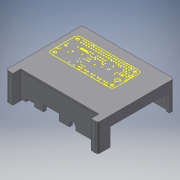
# Autodesk Inventor part: upperPiCase_small
Saved by Autodesk Inventor 2017 (Build 210142000, 142)
## iProperties
Created: 2017-11-29
Part Number: upperPiCase_small
Material: Generic
Document SubType Name: Modeling
Designer: Paolo
Density: 1 g/cm^3
Appearance: Default
Author: Paolo
Autodesk Inventor part; units mm, degrees
ref_plane "YZ Plane" through (0, 0, 0) normal (1, 0, 0) x (0, 1, 0)
ref_plane "XZ Plane" through (0, 0, 0) normal (0, 1, 0) x (-1, 0, 0)
ref_plane "XY Plane" through (0, 0, 0) normal (0, 0, 1) x (1, 0, 0)
ref_plane "Work Plane5" through (0, 0, 0) normal (0, 0, 1) x (1, 0, 0)
sketch "Sketch1" plane through (0, 0, 0) normal (0, 0, 1) x (1, 0, 0)
  line L0 (74.5037, -44.5224) -> (71.3037, -44.5224) projected
  line L1 (71.3037, -44.5224) -> (71.3037, -29.3224) projected
  line L2 (71.3037, -29.3224) -> (74.5037, -29.3224) projected
  line L3 (74.5037, -44.5224) -> (74.5037, -29.3224) projected
  line L4 (74.5037, 13.2776) -> (74.5037, 28.4776) projected
  line L5 (74.5037, 13.2776) -> (71.3037, 13.2776) projected
  line L6 (71.3037, 13.2776) -> (71.3037, 28.4776) projected
  line L7 (71.3037, 28.4776) -> (74.5037, 28.4776) projected
  circle A0 centre (-7.1663, -32.5224) radius 1.1 projected
  line L8 (-11.2963, 13.2776) -> (-14.4963, 13.2776) projected
  line L9 (-14.4963, 28.4776) -> (-14.4963, 13.2776) projected
  line L10 (-14.4963, 28.4776) -> (-11.2963, 28.4776) projected
  line L11 (-11.2963, 28.4776) -> (-11.2963, 13.2776) projected
  line L12 (-11.2963, -44.5224) -> (-14.4963, -44.5224) projected
  line L13 (-14.4963, -29.3224) -> (-14.4963, -44.5224) projected
  line L14 (-14.4963, -29.3224) -> (-11.2963, -29.3224) projected
  line L15 (-11.2963, -29.3224) -> (-11.2963, -44.5224) projected
  circle A1 centre (-7.1663, 16.4776) radius 1.1 projected
  arc A2 (-9.5963, 14.7183) -> (-9.5963, 18.2369) centre (-7.1663, 16.4776) ccw projected
  line L16 (-9.5963, 27.9776) -> (-9.5963, 18.2369) projected
  line L17 (69.6037, 27.9776) -> (-9.5963, 27.9776) projected
  line L18 (69.6037, 27.9776) -> (69.6037, 11.2776) projected
  line L19 (69.6037, 11.2776) -> (71.5037, 11.2776) projected
  line L20 (71.5037, 11.2776) -> (71.5037, -27.3224) projected
  line L21 (71.5037, -27.3224) -> (69.6037, -27.3224) projected
  line L22 (69.6037, -36.0224) -> (69.6037, -27.3224) projected
  line L23 (69.6037, -38.5224) -> (69.6037, -36.0224) projected
  line L24 (69.6037, -46.5224) -> (69.6037, -38.5224) projected
  line L25 (74.5037, -46.5224) -> (69.6037, -46.5224) projected
  arc A3 (74.5037, -46.5224) -> (76.5037, -44.5224) centre (74.5037, -44.5224) ccw projected
  line L26 (76.5037, -44.5224) -> (76.5037, 28.4776) projected
  arc A4 (76.5037, 28.4776) -> (74.5037, 30.4776) centre (74.5037, 28.4776) ccw projected
  line L27 (74.5037, 30.4776) -> (-14.4963, 30.4776) projected
  arc A5 (-14.4963, 30.4776) -> (-16.4963, 28.4776) centre (-14.4963, 28.4776) ccw projected
  line L28 (-16.4963, -44.5224) -> (-16.4963, 28.4776) projected
  arc A6 (-16.4963, -44.5224) -> (-14.4963, -46.5224) centre (-14.4963, -44.5224) ccw projected
  line L29 (-14.4963, -46.5224) -> (-9.5963, -46.5224) projected
  line L30 (-9.5963, -38.5224) -> (-9.5963, -46.5224) projected
  line L31 (-9.5963, -36.0224) -> (-9.5963, -38.5224) projected
  line L32 (-9.5963, -34.2817) -> (-9.5963, -36.0224) projected
  arc A7 (-9.5963, -34.2817) -> (-9.5963, -30.7631) centre (-7.1663, -32.5224) ccw projected
  line L33 (-9.5963, -27.3224) -> (-9.5963, -30.7631) projected
  line L34 (-13.4963, -27.3224) -> (-9.5963, -27.3224) projected
  line L35 (-13.4963, -27.3224) -> (-13.4963, 11.2776) projected
  line L36 (-13.4963, 11.2776) -> (-9.5963, 11.2776) projected
  line L37 (-9.5963, 14.7183) -> (-9.5963, 11.2776) projected
  line L38 (69.6037, -38.5224) -> (-9.5963, -38.5224) projected
  line L39 (-9.5963, -46.5224) -> (69.6037, -46.5224) projected
  point P0 (0, 0)
extrude "Extrusion1" add sketch "Sketch1" along normal blind 2 contours L0 L1 L2 L3 | L5 L6 L7 L4 | A0 | L8 L9 L10 L11 | L12 L13 L14 L15 | A1 | L37 L36 L35 L34 L33 A7 L32 L31 L30 L29 A6 L28 A5 L27 A4 L26 A3 L25 L24 L23 L22 L21 L20 L19 L18 L17 L16 A2 | A2 L16 L17 L18 L19 L20 L21 L22 L23 L38 L31 L32 A7 L33 L34 L35 L36 L37
sketch "Sketch2" plane through (0, 0, 0) normal (0, 0, -1) x (-1, 0, 0)
  line L0 (-69.6037, -38.5224) -> (-69.6037, -46.5224) projected
  line L1 (-69.6037, -46.5224) -> (-74.5037, -46.5224) projected
  arc A0 (-76.5037, -44.5224) -> (-74.5037, -46.5224) centre (-74.5037, -44.5224) ccw projected
  line L2 (-76.5037, -44.5224) -> (-76.5037, 28.4776) projected
  arc A1 (-74.5037, 30.4776) -> (-76.5037, 28.4776) centre (-74.5037, 28.4776) ccw projected
  line L3 (-74.5037, 30.4776) -> (14.4963, 30.4776) projected
  arc A2 (16.4963, 28.4776) -> (14.4963, 30.4776) centre (14.4963, 28.4776) ccw projected
  line L4 (16.4963, 28.4776) -> (16.4963, -44.5224) projected
  arc A3 (14.4963, -46.5224) -> (16.4963, -44.5224) centre (14.4963, -44.5224) ccw projected
  line L5 (14.4963, -46.5224) -> (9.5963, -46.5224) projected
  line L6 (9.5963, -46.5224) -> (9.5963, -38.5224) projected
  line L7 (9.5963, -38.5224) -> (-69.6037, -38.5224) projected
  line L8 (13.4963, -43.5224) -> (13.4963, 27.4776)
  line L9 (13.4963, 27.4776) -> (-73.5037, 27.4776)
  line L10 (-73.5037, 27.4776) -> (-73.5037, -43.5224)
  line L11 (-73.5037, -43.5224) -> (-72.6037, -43.5224)
  line L12 (-72.6037, -43.5224) -> (-72.6037, -35.5224)
  line L13 (-72.6037, -35.5224) -> (12.5963, -35.5224)
  line L14 (12.5963, -35.5224) -> (12.5963, -43.5224)
  line L15 (12.5963, -43.5224) -> (13.4963, -43.5224)
  line L16 (12.5963, -35.5224) -> (13.4963, -35.5224)
  line L17 (-72.6037, -35.5224) -> (-73.5037, -35.5224)
  point P0 (0, 0)
  dimension "d8" = 3
  dimension "d2" = 3
  constraints: 20 end point, 3 point on line, 1 perpendicular, 7 other
  measures "d2" distance between parallel lines of L4 L8
ref_plane "Work Plane2" through (-16.4963, -46.5224, -25.9538) normal (0, 0, 1) x (1, 0, 0)
extrude "Extrusion2" add sketch "Sketch2" along normal up to surface (25.9538 mm away) contours L0 L1 A0 L2 A1 L3 A2 L4 A3 L5 L6 L7 | L15 L14 L16 L8 | L12 L11 L10 L17
ref_plane "Work Plane8" through (76.5037, -44.5224, 2) normal (1, 0, 0) x (0, 0, -1)
sketch "Sketch3" plane through (76.5037, -44.5224, 2) normal (1, 0, 0) x (0, 0, -1)
  line L0 (26.1398, 11) -> (11.52, 11) projected
  line L1 (11.3398, 26.4503) -> (11.3398, 11.0497) projected
  line L2 (26.1398, 26.5) -> (11.52, 26.5) projected
  line L3 (27.9538, 6) -> (27.9538, 6) projected
  line L4 (2, 6) -> (27.9538, 6) projected
  line L5 (2, 6) -> (2, 6) projected
  line L6 (2, 6) -> (27.9538, 6) projected
  line L7 (27.9538, 9) -> (27.9538, 9) projected
  line L8 (2, 9) -> (27.9538, 9) projected
  line L9 (2, 9) -> (2, 9) projected
  line L10 (2, 9) -> (27.9538, 9) projected
  line L11 (2, 72) -> (2, 9) projected
  line L12 (2, 72) -> (27.9538, 72) projected
  line L13 (27.9538, 73) -> (27.9538, 0) projected
  line L14 (27.9538, 10.5) -> (9.8398, 10.5)
  line L15 (9.8398, 10.5) -> (9.8398, 70.5)
  line L16 (9.8398, 70.5) -> (27.9538, 70.5)
  line L17 (27.9538, 70.5) -> (27.9538, 10.5)
  point P0 (2, 44.5224)
  dimension "d5" = 1.5
  dimension "d6" = 1.5
  dimension "d7" = 60
  constraints: 8 end point, 2 parallel, 1 horizontal, 1 perpendicular, 1 point on line
  measures "d5" distance between parallel lines of L8 L14
  measures "d6" distance from line of L1.end L15
  measures "d7" distance between parallel lines of L14 L16
extrude "Extrusion3" cut sketch "Sketch3" against normal blind 3 contours L14 L15 L16 L13
ref_plane "Work Plane7" through (-9.5963, -38.5224, -25.9538) normal (0, -1, 0) x (1, 0, 0)
sketch "Sketch5" plane through (-9.5963, -38.5224, -25.9538) normal (0, -1, 0) x (1, 0, 0)
  circle A0 centre (52.43, 4.6) radius 2.7 projected
  circle A1 centre (52.43, 4.6) radius 3.2
  line L0 (55.63, 4.6) -> (55.63, 0)
  line L1 (83.1, 0) -> (-3.9, 0) projected
  line L2 (49.23, 4.6) -> (49.23, 0)
  line L3 (49.23, 0) -> (55.63, 0)
  point P0 (9.5963, 25.9538)
  dimension "d10" = 0.5
  constraints: 6 end point, 2 point on circle, 2 tangent, 1 centre point, 1 parallel, 1 perpendicular, 1 point on line, 1 vertical
  measures "d10" radial gap between concentric circles of A0 A1
extrude "Extrusion4" cut sketch "Sketch5" against normal blind 3 contours A0 | A1 | L0 L1 L2 A1
sketch "Sketch6" plane through (-9.5963, -38.5224, 0) normal (0, -1, 0) x (1, 0, 0)
  line L0 (79.2, -24.3538) -> (0, -24.3538) projected
  line L1 (0, -25.9538) -> (0, -24.3538) projected
  line L2 (0, -33.9538) -> (0, -25.9538) projected
  line L3 (79.2, -33.9538) -> (0, -33.9538) projected
  line L4 (79.2, -25.9538) -> (79.2, -33.9538) projected
  line L5 (79.2, -25.9538) -> (79.2, -24.3538) projected
  line L6 (0, -25.9538) -> (79.2, -25.9538)
  line L7 (79.2, -25.9538) -> (79.2, -24.3538)
  line L8 (79.2, -24.3538) -> (0, -24.3538)
  line L9 (0, -24.3538) -> (0, -25.9538)
  point P0 (9.5963, 0)
  constraints: 8 end point, 2 parallel, 1 horizontal, 1 perpendicular
extrude "Extrusion5" cut sketch "Sketch6" against normal blind 3 contours L5 L6 L1 L0
ref_plane "Work Plane6" through (-9.5963, -38.5224, 0) normal (0, -1, 0) x (1, 0, 0)
sketch "Sketch7" plane through (-9.5963, -38.5224, 0) normal (0, -1, 0) x (1, 0, 0)
  line L0 (38.43, -21.5238) -> (38.43, -23.6238) projected
  line L1 (23.43, -23.6238) -> (23.43, -21.5238) projected
  line L2 (13.28, -23.0667) -> (13.28, -22.4238) projected
  line L3 (12.73, -21.8738) -> (11.8185, -21.8738) projected
  line L4 (7.2415, -21.8738) -> (6.33, -21.8738) projected
  line L5 (5.78, -22.4238) -> (5.78, -23.0667) projected
  line L6 (33.05, -18.2738) -> (28.81, -18.2738) projected
  line L7 (0, -24.3538) -> (49.23, -24.3538) projected
  line L8 (5.28, -24.3538) -> (13.78, -24.3538)
  line L9 (13.78, -24.3538) -> (13.78, -21.3738)
  line L10 (13.78, -21.3738) -> (5.28, -21.3738)
  line L11 (5.28, -21.3738) -> (5.28, -24.3538)
  line L12 (22.93, -24.3538) -> (38.93, -24.3538)
  line L13 (38.93, -24.3538) -> (38.93, -17.7738)
  line L14 (38.93, -17.7738) -> (22.93, -17.7738)
  line L15 (22.93, -17.7738) -> (22.93, -24.3538)
  point P0 (9.5963, 0)
  dimension "d15" = 0.5
  dimension "d16" = 0.5
  dimension "d17" = 0.5
  dimension "d18" = 0.5
  dimension "d19" = 0.5
  dimension "d20" = 0.5
  constraints: 16 end point, 4 parallel, 2 horizontal, 2 perpendicular, 2 point on line
  measures "d15" distance between parallel lines of L11 L5
  measures "d16" distance between parallel lines of L9 L2
  measures "d17" distance between parallel lines of L10 L4
  measures "d18" distance between parallel lines of L15 L1
  measures "d19" distance between parallel lines of L13 L0
  measures "d20" distance between parallel lines of L14 L6
extrude "Extrusion6" cut sketch "Sketch7" against normal blind 3
sketch "Sketch8" plane through (0, 0, 2) normal (0, 0, 1) x (1, 0, 0)
  arc A0 (51.3247, -10.0244) -> (54.3247, -7.0244) centre (51.3247, -7.0244) ccw projected
  line L0 (51.3247, -10.0244) -> (-7.6753, -10.0244) projected
  arc A1 (-10.6753, -7.0244) -> (-7.6753, -10.0244) centre (-7.6753, -7.0244) ccw projected
  line L1 (-10.6753, -7.0244) -> (-10.6753, 16.9756) projected
  arc A2 (-7.6753, 19.9756) -> (-10.6753, 16.9756) centre (-7.6753, 16.9756) ccw projected
  line L2 (-7.6753, 19.9756) -> (51.3247, 19.9756) projected
  arc A3 (54.3247, 16.9756) -> (51.3247, 19.9756) centre (51.3247, 16.9756) ccw projected
  line L3 (54.3247, 16.9756) -> (54.3247, -7.0244) projected
  circle A4 centre (-7.6753, -0.5244) radius 0.1651 projected
  circle A5 centre (11.5247, 0.0756) radius 0.1651 projected
  circle A6 centre (12.4597, -3.3894) radius 0.1651 projected
  circle A7 centre (51.5747, 1.4074) radius 0.1651 projected
  circle A8 centre (49.8747, 2.4256) radius 0.1651 projected
  circle A9 centre (50.8247, 7.5006) radius 0.1651 projected
  circle A10 centre (46.8247, 7.9756) radius 0.1651 projected
  circle A11 centre (50.8247, 10.4756) radius 0.1651 projected
  circle A12 centre (34.8247, 4.9756) radius 0.1651 projected
  circle A13 centre (34.8247, 10.9756) radius 0.1651 projected
  circle A14 centre (0.9247, 3.2756) radius 0.1651 projected
  circle A15 centre (50.8247, 8.4756) radius 0.1651 projected
  circle A16 centre (35.3647, 9.9356) radius 0.1651 projected
  circle A17 centre (35.8247, 5.9756) radius 0.1651 projected
  circle A18 centre (1.9247, 3.2756) radius 0.1651 projected
  circle A19 centre (3.1247, 10.4756) radius 0.1651 projected
  circle A20 centre (4.1247, 10.4756) radius 0.1651 projected
  circle A21 centre (5.1247, 10.4756) radius 0.1651 projected
  circle A22 centre (6.1247, 10.4756) radius 0.1651 projected
  circle A23 centre (7.1247, 10.4756) radius 0.1651 projected
  circle A24 centre (8.1247, 10.4756) radius 0.1651 projected
  circle A25 centre (9.1247, 10.4756) radius 0.1651 projected
  circle A26 centre (3.1247, 9.4756) radius 0.1651 projected
  circle A27 centre (4.1247, 9.4756) radius 0.1651 projected
  circle A28 centre (5.1247, 9.4756) radius 0.1651 projected
  circle A29 centre (6.1247, 9.4756) radius 0.1651 projected
  circle A30 centre (7.1247, 9.4756) radius 0.1651 projected
  circle A31 centre (8.1247, 9.4756) radius 0.1651 projected
  circle A32 centre (9.1247, 9.4756) radius 0.1651 projected
  circle A33 centre (8.8247, 4.9756) radius 0.1651 projected
  circle A34 centre (18.5247, 2.5756) radius 0.1651 projected
  circle A35 centre (24.2247, 2.5756) radius 0.1651 projected
  circle A36 centre (44.8247, 18.5756) radius 0.1651 projected
  circle A37 centre (6.6247, 19.0756) radius 0.1651 projected
  circle A38 centre (47.2247, 16.6836) radius 0.1651 projected
  circle A39 centre (37.6247, 13.2756) radius 0.1651 projected
  circle A40 centre (26.8247, 6.9756) radius 0.1651 projected
  circle A41 centre (15.3247, 2.2756) radius 0.1651 projected
  circle A42 centre (14.6247, -2.0244) radius 0.1651 projected
  circle A43 centre (8.9247, -8.0244) radius 0.1651 projected
  circle A44 centre (49.8747, -2.5744) radius 0.1651 projected
  circle A45 centre (53.6247, 3.6074) radius 0.1651 projected
  circle A46 centre (53.6032, 5.0972) radius 0.1651 projected
  circle A47 centre (53.623, 6.8074) radius 0.1651 projected
  circle A48 centre (52.5247, 12.1574) radius 0.1651 projected
  circle A49 centre (42.6297, 6.8706) radius 0.1651 projected
  circle A50 centre (39.5747, 13.5256) radius 0.1651 projected
  circle A51 centre (39.5747, 19.6256) radius 0.1651 projected
  circle A52 centre (52.5247, 13.3756) radius 0.1651 projected
  circle A53 centre (53.1747, 9.0256) radius 0.1651 projected
  circle A54 centre (13.5247, 2.1074) radius 0.1651 projected
  circle A55 centre (0.3247, 9.5756) radius 0.1651 projected
  circle A56 centre (48.9247, 12.8756) radius 0.1651 projected
  circle A57 centre (20.2247, -9.4244) radius 0.1651 projected
  circle A58 centre (-9.6753, -1.8244) radius 0.1651 projected
  circle A59 centre (-8.6753, -1.8244) radius 0.1651 projected
  circle A60 centre (-8.0753, 7.2756) radius 0.1651 projected
  circle A61 centre (26.6247, -9.4244) radius 0.1651 projected
  circle A62 centre (33.1247, -9.4244) radius 0.1651 projected
  circle A63 centre (39.5247, -9.4244) radius 0.1651 projected
  circle A64 centre (45.9247, -9.4244) radius 0.1651 projected
  circle A65 centre (17.1247, 2.5756) radius 0.1651 projected
  circle A66 centre (28.6247, 6.9756) radius 0.1651 projected
  circle A67 centre (28.6247, 8.7756) radius 0.1651 projected
  circle A68 centre (29.4247, 14.4756) radius 0.1651 projected
  circle A69 centre (48.0247, 18.2756) radius 0.1651 projected
  circle A70 centre (42.5247, 4.4756) radius 0.1651 projected
  circle A71 centre (29.7247, 4.2756) radius 0.1651 projected
  circle A72 centre (48.0247, -9.3244) radius 0.1651 projected
  circle A73 centre (15.6247, 7.5756) radius 0.1651 projected
  circle A74 centre (19.8247, 7.5756) radius 0.1651 projected
  circle A75 centre (19.0881, 7.5756) radius 0.1651 projected
  circle A76 centre (16.3613, 7.5756) radius 0.1651 projected
  circle A77 centre (18.0147, 9.2056) radius 0.5 projected
  circle A78 centre (25.6347, 9.2056) radius 0.5 projected
  circle A79 centre (18.0147, 11.7456) radius 0.5 projected
  circle A80 centre (25.6347, 11.7456) radius 0.5 projected
  circle A81 centre (23.0947, 11.7456) radius 0.5 projected
  circle A82 centre (23.0947, 9.2056) radius 0.5 projected
  circle A83 centre (20.5547, 11.7456) radius 0.5 projected
  circle A84 centre (20.5547, 9.2056) radius 0.5 projected
  circle A85 centre (17.7247, -7.0244) radius 0.5999 projected
  circle A86 centre (20.2647, -7.0244) radius 0.5999 projected
  circle A87 centre (24.1247, -7.0244) radius 0.5999 projected
  circle A88 centre (26.6647, -7.0244) radius 0.5999 projected
  circle A89 centre (30.5247, -7.0244) radius 0.5999 projected
  circle A90 centre (33.0647, -7.0244) radius 0.5999 projected
  circle A91 centre (36.9247, -7.0244) radius 0.5999 projected
  circle A92 centre (39.4647, -7.0244) radius 0.5999 projected
  circle A93 centre (43.3247, -7.0244) radius 0.5999 projected
  circle A94 centre (45.8647, -7.0244) radius 0.5999 projected
  circle A95 centre (10.8247, 8.9756) radius 0.4064 projected
  circle A96 centre (13.3247, 8.9756) radius 0.4064 projected
  circle A97 centre (13.3247, 11.4756) radius 0.4064 projected
  circle A98 centre (10.8247, 11.4756) radius 0.4064 projected
  circle A99 centre (14.8247, 4.9756) radius 0.4064 projected
  circle A100 centre (17.3247, 4.9756) radius 0.4064 projected
  circle A101 centre (13.8247, -8.5244) radius 0.4064 projected
  circle A102 centre (45.9247, 12.5756) radius 0.4064 projected
  circle A103 centre (43.4247, 12.5756) radius 0.4064 projected
  circle A104 centre (45.9547, 17.7456) radius 0.5 projected
  circle A105 centre (-2.3053, 17.7456) radius 0.5 projected
  circle A106 centre (45.9547, 15.2056) radius 0.5 projected
  circle A107 centre (-2.3053, 15.2056) radius 0.5 projected
  circle A108 centre (0.2347, 15.2056) radius 0.5 projected
  circle A109 centre (0.2347, 17.7456) radius 0.5 projected
  circle A110 centre (2.7747, 15.2056) radius 0.5 projected
  circle A111 centre (2.7747, 17.7456) radius 0.5 projected
  circle A112 centre (5.3147, 15.2056) radius 0.5 projected
  circle A113 centre (5.3147, 17.7456) radius 0.5 projected
  circle A114 centre (7.8547, 15.2056) radius 0.5 projected
  circle A115 centre (7.8547, 17.7456) radius 0.5 projected
  circle A116 centre (10.3947, 15.2056) radius 0.5 projected
  circle A117 centre (10.3947, 17.7456) radius 0.5 projected
  circle A118 centre (12.9347, 15.2056) radius 0.5 projected
  circle A119 centre (12.9347, 17.7456) radius 0.5 projected
  circle A120 centre (15.4747, 15.2056) radius 0.5 projected
  circle A121 centre (15.4747, 17.7456) radius 0.5 projected
  circle A122 centre (18.0147, 15.2056) radius 0.5 projected
  circle A123 centre (18.0147, 17.7456) radius 0.5 projected
  circle A124 centre (20.5547, 15.2056) radius 0.5 projected
  circle A125 centre (20.5547, 17.7456) radius 0.5 projected
  circle A126 centre (23.0947, 15.2056) radius 0.5 projected
  circle A127 centre (23.0947, 17.7456) radius 0.5 projected
  circle A128 centre (25.6347, 15.2056) radius 0.5 projected
  circle A129 centre (25.6347, 17.7456) radius 0.5 projected
  circle A130 centre (28.1747, 15.2056) radius 0.5 projected
  circle A131 centre (28.1747, 17.7456) radius 0.5 projected
  circle A132 centre (30.7147, 15.2056) radius 0.5 projected
  circle A133 centre (30.7147, 17.7456) radius 0.5 projected
  circle A134 centre (33.2547, 15.2056) radius 0.5 projected
  circle A135 centre (33.2547, 17.7456) radius 0.5 projected
  circle A136 centre (35.7947, 15.2056) radius 0.5 projected
  circle A137 centre (35.7947, 17.7456) radius 0.5 projected
  circle A138 centre (38.3347, 15.2056) radius 0.5 projected
  circle A139 centre (38.3347, 17.7456) radius 0.5 projected
  circle A140 centre (40.8747, 15.2056) radius 0.5 projected
  circle A141 centre (40.8747, 17.7456) radius 0.5 projected
  circle A142 centre (43.4147, 15.2056) radius 0.5 projected
  circle A143 centre (43.4147, 17.7456) radius 0.5 projected
  circle A144 centre (-7.6753, 4.9756) radius 0.9 projected
  circle A145 centre (50.8247, 16.4756) radius 1.397 projected
  circle A146 centre (50.8247, -6.5244) radius 1.397 projected
  circle A147 centre (-7.1753, 16.4756) radius 1.397 projected
  circle A148 centre (-7.1753, -6.5244) radius 1.397 projected
  circle A149 centre (48.9247, 0.4756) radius 2.1 projected
  line L4 (51.3247, 11.3756) -> (51.3247, 9.3756) projected
  line L5 (51.3247, 9.3756) -> (53.7247, 9.3756) projected
  line L6 (53.7247, 9.3756) -> (53.7247, 11.3756) projected
  line L7 (53.7247, 11.3756) -> (51.3247, 11.3756) projected
  circle A150 centre (51.8747, 9.5756) radius 0.075 projected
  line L8 (48.1259, 11.0768) -> (44.5235, 11.0768) projected
  line L9 (44.5235, 11.0768) -> (44.5235, 6.4744) projected
  line L10 (44.5235, 6.4744) -> (48.1259, 6.4744) projected
  line L11 (48.1259, 6.4744) -> (48.1259, 11.0768) projected
  circle A151 centre (47.4947, 7.1056) radius 0.3377 projected
  line L12 (19.4247, -9.9244) -> (19.4247, -9.9244) projected
  line L13 (21.1047, -9.9244) -> (19.4247, -9.9244) projected
  line L14 (21.1047, -9.9244) -> (21.1047, -9.9244) projected
  line L15 (21.1047, -9.9244) -> (21.5347, -9.9244) projected
  line L16 (21.5347, -9.9244) -> (21.5347, -9.9244) projected
  line L17 (16.4547, -9.9244) -> (21.5347, -9.9244) projected
  line L18 (16.4547, -9.9244) -> (16.4547, -9.9244) projected
  line L19 (16.4547, -9.9244) -> (16.8847, -9.9244) projected
  line L20 (16.8847, -9.9244) -> (16.8847, -9.9244) projected
  line L21 (18.5647, -9.9244) -> (16.8847, -9.9244) projected
  line L22 (18.5647, -9.9244) -> (18.5647, -9.9244) projected
  line L23 (18.5647, -9.9244) -> (19.4247, -9.9244) projected
  line L24 (19.4247, -4.1244) -> (19.4247, -4.1244) projected
  line L25 (18.5647, -4.1244) -> (19.4247, -4.1244) projected
  line L26 (18.5647, -4.1244) -> (18.5647, -4.1244) projected
  line L27 (18.5647, -4.1244) -> (16.8847, -4.1244) projected
  line L28 (16.8847, -4.1244) -> (16.8847, -4.1244) projected
  line L29 (16.4547, -4.1244) -> (16.8847, -4.1244) projected
  line L30 (16.4547, -4.1244) -> (16.4547, -4.1244) projected
  line L31 (16.4547, -4.1244) -> (17.7247, -4.1244) projected
  line L32 (17.7247, -4.1244) -> (17.7247, -4.1244) projected
  line L33 (17.7247, -4.1244) -> (17.9977, -4.1244) projected
  line L34 (17.9977, -4.1244) -> (19.9917, -4.1244) projected
  line L35 (19.9917, -4.1244) -> (20.2647, -4.1244) projected
  line L36 (20.2647, -4.1244) -> (20.2647, -4.1244) projected
  line L37 (20.2647, -4.1244) -> (21.5347, -4.1244) projected
  line L38 (21.5347, -4.1244) -> (21.5347, -4.1244) projected
  line L39 (21.1047, -4.1244) -> (21.5347, -4.1244) projected
  line L40 (21.1047, -4.1244) -> (21.1047, -4.1244) projected
  line L41 (21.1047, -4.1244) -> (19.4247, -4.1244) projected
  line L42 (25.8247, -9.9244) -> (25.8247, -9.9244) projected
  line L43 (27.5047, -9.9244) -> (25.8247, -9.9244) projected
  line L44 (27.5047, -9.9244) -> (27.5047, -9.9244) projected
  line L45 (27.5047, -9.9244) -> (27.9347, -9.9244) projected
  line L46 (27.9347, -9.9244) -> (27.9347, -9.9244) projected
  line L47 (22.8547, -9.9244) -> (27.9347, -9.9244) projected
  line L48 (22.8547, -9.9244) -> (22.8547, -9.9244) projected
  line L49 (22.8547, -9.9244) -> (23.2847, -9.9244) projected
  line L50 (23.2847, -9.9244) -> (23.2847, -9.9244) projected
  line L51 (24.9647, -9.9244) -> (23.2847, -9.9244) projected
  line L52 (24.9647, -9.9244) -> (24.9647, -9.9244) projected
  line L53 (24.9647, -9.9244) -> (25.8247, -9.9244) projected
  line L54 (43.3247, -4.1244) -> (43.3247, -5.7244) projected
  line L55 (42.0547, -4.1244) -> (43.3247, -4.1244) projected
  line L56 (42.0547, -4.1244) -> (42.0547, -9.9244) projected
  line L57 (42.0547, -9.9244) -> (47.1347, -9.9244) projected
  line L58 (47.1347, -4.1244) -> (47.1347, -9.9244) projected
  line L59 (45.8647, -4.1244) -> (47.1347, -4.1244) projected
  line L60 (45.8647, -4.1244) -> (45.8647, -5.7244) projected
  line L61 (43.3247, -5.7244) -> (45.8647, -5.7244) projected
  line L62 (43.0047, -7.3244) -> (43.0047, -6.6844) projected
  line L63 (43.0047, -6.6844) -> (43.6447, -6.6844) projected
  line L64 (43.6447, -7.3244) -> (43.6447, -6.6844) projected
  line L65 (43.0047, -7.3244) -> (43.6447, -7.3244) projected
  line L66 (45.5447, -7.3244) -> (45.5447, -6.6844) projected
  line L67 (45.5447, -6.6844) -> (46.1847, -6.6844) projected
  line L68 (46.1847, -7.3244) -> (46.1847, -6.6844) projected
  line L69 (45.5447, -7.3244) -> (46.1847, -7.3244) projected
  line L70 (44.2897, -6.2544) -> (44.2897, -7.7544) projected
  line L71 (44.8997, -6.2544) -> (44.2897, -6.2544) projected
  line L72 (44.8997, -7.7544) -> (44.8997, -6.2544) projected
  line L73 (44.2897, -7.7544) -> (44.8997, -7.7544) projected
  line L74 (36.9247, -4.1244) -> (36.9247, -5.7244) projected
  line L75 (35.6547, -4.1244) -> (36.9247, -4.1244) projected
  line L76 (35.6547, -4.1244) -> (35.6547, -9.9244) projected
  line L77 (35.6547, -9.9244) -> (40.7347, -9.9244) projected
  line L78 (40.7347, -4.1244) -> (40.7347, -9.9244) projected
  line L79 (39.4647, -4.1244) -> (40.7347, -4.1244) projected
  line L80 (39.4647, -4.1244) -> (39.4647, -5.7244) projected
  line L81 (36.9247, -5.7244) -> (39.4647, -5.7244) projected
  line L82 (36.6047, -7.3244) -> (36.6047, -6.6844) projected
  line L83 (36.6047, -6.6844) -> (37.2447, -6.6844) projected
  line L84 (37.2447, -7.3244) -> (37.2447, -6.6844) projected
  line L85 (36.6047, -7.3244) -> (37.2447, -7.3244) projected
  line L86 (39.1447, -7.3244) -> (39.1447, -6.6844) projected
  line L87 (39.1447, -6.6844) -> (39.7847, -6.6844) projected
  line L88 (39.7847, -7.3244) -> (39.7847, -6.6844) projected
  line L89 (39.1447, -7.3244) -> (39.7847, -7.3244) projected
  line L90 (37.8897, -6.2544) -> (37.8897, -7.7544) projected
  line L91 (38.4997, -6.2544) -> (37.8897, -6.2544) projected
  line L92 (38.4997, -7.7544) -> (38.4997, -6.2544) projected
  line L93 (37.8897, -7.7544) -> (38.4997, -7.7544) projected
  line L94 (30.5247, -4.1244) -> (30.5247, -5.7244) projected
  line L95 (29.2547, -4.1244) -> (30.5247, -4.1244) projected
  line L96 (29.2547, -4.1244) -> (29.2547, -9.9244) projected
  line L97 (29.2547, -9.9244) -> (34.3347, -9.9244) projected
  line L98 (34.3347, -4.1244) -> (34.3347, -9.9244) projected
  line L99 (33.0647, -4.1244) -> (34.3347, -4.1244) projected
  line L100 (33.0647, -4.1244) -> (33.0647, -5.7244) projected
  line L101 (30.5247, -5.7244) -> (33.0647, -5.7244) projected
  line L102 (30.2047, -7.3244) -> (30.2047, -6.6844) projected
  line L103 (30.2047, -6.6844) -> (30.8447, -6.6844) projected
  line L104 (30.8447, -7.3244) -> (30.8447, -6.6844) projected
  line L105 (30.2047, -7.3244) -> (30.8447, -7.3244) projected
  line L106 (32.7447, -7.3244) -> (32.7447, -6.6844) projected
  line L107 (32.7447, -6.6844) -> (33.3847, -6.6844) projected
  line L108 (33.3847, -7.3244) -> (33.3847, -6.6844) projected
  line L109 (32.7447, -7.3244) -> (33.3847, -7.3244) projected
  line L110 (31.4897, -6.2544) -> (31.4897, -7.7544) projected
  line L111 (32.0997, -6.2544) -> (31.4897, -6.2544) projected
  line L112 (32.0997, -7.7544) -> (32.0997, -6.2544) projected
  line L113 (31.4897, -7.7544) -> (32.0997, -7.7544) projected
  line L114 (24.1247, -4.1244) -> (24.1247, -5.7244) projected
  line L115 (22.8547, -4.1244) -> (24.1247, -4.1244) projected
  line L116 (22.8547, -4.1244) -> (22.8547, -9.9244) projected
  line L117 (22.8547, -9.9244) -> (27.9347, -9.9244) projected
  line L118 (27.9347, -4.1244) -> (27.9347, -9.9244) projected
  line L119 (26.6647, -4.1244) -> (27.9347, -4.1244) projected
  line L120 (26.6647, -4.1244) -> (26.6647, -5.7244) projected
  line L121 (24.1247, -5.7244) -> (26.6647, -5.7244) projected
  line L122 (23.8047, -7.3244) -> (23.8047, -6.6844) projected
  line L123 (23.8047, -6.6844) -> (24.4447, -6.6844) projected
  line L124 (24.4447, -7.3244) -> (24.4447, -6.6844) projected
  line L125 (23.8047, -7.3244) -> (24.4447, -7.3244) projected
  line L126 (26.3447, -7.3244) -> (26.3447, -6.6844) projected
  line L127 (26.3447, -6.6844) -> (26.9847, -6.6844) projected
  line L128 (26.9847, -7.3244) -> (26.9847, -6.6844) projected
  line L129 (26.3447, -7.3244) -> (26.9847, -7.3244) projected
  line L130 (25.0897, -6.2544) -> (25.0897, -7.7544) projected
  line L131 (25.6997, -6.2544) -> (25.0897, -6.2544) projected
  line L132 (25.6997, -7.7544) -> (25.6997, -6.2544) projected
  line L133 (25.0897, -7.7544) -> (25.6997, -7.7544) projected
  line L134 (17.7247, -4.1244) -> (17.7247, -5.7244) projected
  line L135 (16.4547, -4.1244) -> (17.7247, -4.1244) projected
  line L136 (16.4547, -4.1244) -> (16.4547, -9.9244) projected
  line L137 (16.4547, -9.9244) -> (21.5347, -9.9244) projected
  line L138 (21.5347, -4.1244) -> (21.5347, -9.9244) projected
  line L139 (20.2647, -4.1244) -> (21.5347, -4.1244) projected
  line L140 (20.2647, -4.1244) -> (20.2647, -5.7244) projected
  line L141 (17.7247, -5.7244) -> (20.2647, -5.7244) projected
  line L142 (17.4047, -7.3244) -> (17.4047, -6.6844) projected
  line L143 (17.4047, -6.6844) -> (18.0447, -6.6844) projected
  line L144 (18.0447, -7.3244) -> (18.0447, -6.6844) projected
  line L145 (17.4047, -7.3244) -> (18.0447, -7.3244) projected
  line L146 (19.9447, -7.3244) -> (19.9447, -6.6844) projected
  line L147 (19.9447, -6.6844) -> (20.5847, -6.6844) projected
  line L148 (20.5847, -7.3244) -> (20.5847, -6.6844) projected
  line L149 (19.9447, -7.3244) -> (20.5847, -7.3244) projected
  line L150 (18.6897, -6.2544) -> (18.6897, -7.7544) projected
  line L151 (19.2997, -6.2544) -> (18.6897, -6.2544) projected
  line L152 (19.2997, -7.7544) -> (19.2997, -6.2544) projected
  line L153 (18.6897, -7.7544) -> (19.2997, -7.7544) projected
  line L154 (14.9547, -2.6244) -> (48.6347, -2.6244)
  line L155 (48.6347, -2.6244) -> (48.6347, -11.5244)
  line L156 (48.6347, -11.5244) -> (14.9547, -11.5244)
  line L157 (14.9547, -11.5244) -> (14.9547, -2.6244)
  line L158 (54.3247, 14.5032) -> (46.4997, 14.5032)
  line L159 (46.4997, 14.5032) -> (46.4997, 5.3226)
  line L160 (46.4997, 5.3226) -> (54.3247, 5.3226)
  line L161 (54.3247, 5.3226) -> (54.3247, 14.5032)
  point P0 (0, 0)
  dimension "d23" = 1.5
  dimension "d24" = 1.5
  dimension "d25" = 1.5
  dimension "d26" = 1.5
  constraints: 16 end point, 4 parallel, 2 horizontal, 2 perpendicular, 1 point on line
  measures "d23" distance from line of L156.end L0
  measures "d24" distance from line of L156.end L136
  measures "d25" distance from line of L154.start L29
  measures "d26" distance from line of L154.end L58
extrude "Extrusion7" cut sketch "Sketch8" against normal blind 3 contours L155 L156 L157 L0 | L0 L157 L154 L155 | L160 L159 L10 L11 L8 L158 L3 | L159 L8 L11 L10 | A9 | A10 | A11 | A15 | A47 | A48 | A52 | A53 | A56 | A57 | A61 | A62 | A63 | A64 | A72 | A85 | A86 | A87 | A88 | A89 | A90 | A91 | A92 | A93 | A94 | L7 L6 L5 L4 | A150 | A151 | L13 L17 L136 L29 L27 L134 L141 L140 L37 L138 L15 | L140 L141 L134 L27 L25 L34 L35 | L43 L47 L116 L115 L114 L121 L120 L119 L118 L45 | L54 L61 L60 L59 L58 L57 L56 L55 | L62 L63 L64 L65 | L66 L67 L68 L69 | L71 L72 L73 L70 | L74 L81 L80 L79 L78 L77 L76 L75 | L82 L83 L84 L85 | L86 L87 L88 L89 | L91 L92 L93 L90 | L94 L101 L100 L99 L98 L97 L96 L95 | L102 L103 L104 L105 | L106 L107 L108 L109 | L111 L112 L113 L110 | L122 L123 L124 L125 | L126 L127 L128 L129 | L131 L132 L133 L130 | L142 L143 L144 L145 | L146 L147 L148 L149 | L151 L152 L153 L150
sketch "Sketch9" plane through (-16.4963, -44.5224, 2) normal (-1, 0, 0) x (0, 0, 1)
  circle A0 centre (-7.4958, 49.198) radius 3.1496 projected
  circle A1 centre (-7.4958, 49.198) radius 5.1496
  point P0 (-2, 44.5224)
  dimension "d29" = 2
  constraints: 1 centre point
  measures "d29" radial gap between concentric circles of A0 A1
extrude "Extrusion8" cut sketch "Sketch9" against normal blind 3 contours A0 | A1
body "Solid1"
